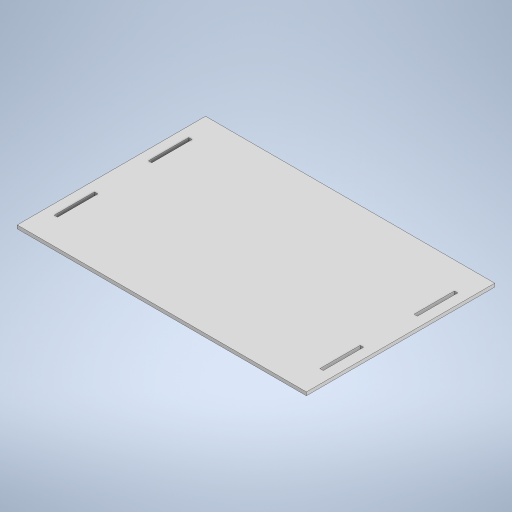
# Autodesk Inventor part: C4Base
Saved by Autodesk Inventor 2024 (Build 280153000, 153)
## iProperties
Created: 2023-11-07
Part Number: C4Base
Material: Generic
Document SubType Name: Modeling
Designer: flynf
Density: 1 g/cm^3
Appearance: Default
Author: flynf
Autodesk Inventor part; units mm, degrees
ref_plane "YZ Plane" through (0, 0, 0) normal (1, 0, 0) x (0, 1, 0)
ref_plane "XZ Plane" through (0, 0, 0) normal (0, 1, 0) x (-1, 0, 0)
ref_plane "XY Plane" through (0, 0, 0) normal (0, 0, 1) x (1, 0, 0)
sketch "Sketch1" plane through (0, 0, 0) normal (0, 1, 0) x (-1, 0, 0)
  line L0 (0, 0) -> (-273.05, 0)
  line L1 (-273.05, 0) -> (-273.05, -177.8)
  line L2 (-273.05, -177.8) -> (0, -177.8)
  line L3 (0, -177.8) -> (0, 0)
  line L4 (-260.35, -25.4) -> (-263.525, -25.4)
  line L5 (-263.525, -25.4) -> (-263.525, -63.5)
  line L6 (-263.525, -63.5) -> (-260.35, -63.5)
  line L7 (-260.35, -63.5) -> (-260.35, -25.4)
  line L8 (-260.35, -114.3) -> (-263.525, -114.3)
  line L9 (-263.525, -114.3) -> (-263.525, -152.4)
  line L10 (-263.525, -152.4) -> (-260.35, -152.4)
  line L11 (-260.35, -152.4) -> (-260.35, -114.3)
  line L12 (-9.525, -25.4) -> (-12.7, -25.4)
  line L13 (-12.7, -25.4) -> (-12.7, -63.5)
  line L14 (-12.7, -63.5) -> (-9.525, -63.5)
  line L15 (-9.525, -63.5) -> (-9.525, -25.4)
  line L16 (-9.525, -114.3) -> (-12.7, -114.3)
  line L17 (-12.7, -114.3) -> (-12.7, -152.4)
  line L18 (-12.7, -152.4) -> (-9.525, -152.4)
  line L19 (-9.525, -152.4) -> (-9.525, -114.3)
  dimension "d0" = 273.05
  dimension "d1" = 177.8
  dimension "d2" = 3.175
  dimension "d3" = 3.175
  dimension "d4" = 3.175
  dimension "d5" = 3.175
  dimension "d6" = 9.525
  dimension "d7" = 9.525
  dimension "d8" = 38.1
  dimension "d9" = 38.1
  dimension "d10" = 38.1
  dimension "d11" = 38.1
  dimension "d12" = 9.525
  dimension "d13" = 9.525
  dimension "d14" = 25.4
  dimension "d15" = 25.4
  dimension "d16" = 25.4
  dimension "d17" = 25.4
  constraints: 40 end point, 10 parallel, 5 horizontal, 5 perpendicular
  measures "d0" distance of L2.end L1.end
  measures "d1" distance of L0.end L1.end
  measures "d2" distance of L9.end L10.end
  measures "d3" distance of L5.end L6.end
  measures "d4" distance of L13.end L14.end
  measures "d5" distance of L17.end L18.end
  measures "d6" distance between parallel lines of L1 L9
  measures "d7" distance between parallel lines of L1 L5
  measures "d8" distance of L6.end L4.start
  measures "d9" distance of L10.end L8.start
  measures "d10" distance of L18.end L16.start
  measures "d11" distance of L14.end L12.start
  measures "d12" distance between parallel lines of L3 L15
  measures "d13" distance between parallel lines of L3 L19
  measures "d14" distance between parallel lines of L2 L10
  measures "d15" distance between parallel lines of L0 L4
  measures "d16" distance between parallel lines of L0 L12
  measures "d17" distance between parallel lines of L2 L18
extrude "Extrusion1" add sketch "Sketch1" along normal blind 3.175
body "Solid1"
